Autodesk Fusion 360 part; units mm, degrees
(part 5 of 5)
  spline S157 degree 5 poles (17.2538, -21.1174) (17.2562, -21.1195) (17.2652, -21.1272) (17.281, -21.1406) (17.3036, -21.1597) (17.333, -21.1842) (17.3671, -21.2121) (17.4015, -21.2398) (17.4361, -21.2672) (17.4709, -21.2944) (17.506, -21.3214) (17.5413, -21.3481) (17.5769, -21.3747) (17.6126, -21.401) (17.6486, -21.4271) (17.6847, -21.4531) (17.7211, -21.4788) (17.7577, -21.5044) (17.7944, -21.5297) (17.8313, -21.5549) (17.8685, -21.5799) (17.9058, -21.6047) (17.9432, -21.6293) (17.9809, -21.6538) (18.0187, -21.6781) (18.0567, -21.7022) (18.0948, -21.7261) (18.1331, -21.7499) (18.1716, -21.7735) (18.2102, -21.7969) (18.249, -21.8202) (18.288, -21.8433) (18.3271, -21.8662) (18.3663, -21.889) (18.4057, -21.9116) (18.4452, -21.9341) (18.4849, -21.9564) (18.5247, -21.9785) (18.5646, -22.0005) (18.6047, -22.0224) (18.645, -22.0441) (18.6853, -22.0656) (18.7258, -22.087) (18.7664, -22.1083) (18.8072, -22.1294) (18.8481, -22.1503) (18.8891, -22.1711) (18.9302, -22.1918) (18.9715, -22.2123) (19.0129, -22.2326) (19.0544, -22.2529) (19.096, -22.2729) (19.1378, -22.2929) (19.1797, -22.3127) (19.2217, -22.3323) (19.2638, -22.3518) (19.306, -22.3712) (19.3483, -22.3904) (19.3908, -22.4095) (19.4334, -22.4284) (19.476, -22.4473) (19.5188, -22.4659) (19.5531, -22.4808) (19.5789, -22.4918) (19.5961, -22.4992) (19.6048, -22.5028) knots 0.13777296 0.13777296 0.13777296 0.13777296 0.13777296 0.13777296 0.14285714 0.15714286 0.17142857 0.18571429 0.2 0.21428571 0.22857143 0.24285714 0.25714286 0.27142857 0.28571429 0.3 0.31428571 0.32857143 0.34285714 0.35714286 0.37142857 0.38571429 0.4 0.41428571 0.42857143 0.44285714 0.45714286 0.47142857 0.48571429 0.5 0.51428571 0.52857143 0.54285714 0.55714286 0.57142857 0.58571429 0.6 0.61428571 0.62857143 0.64285714 0.65714286 0.67142857 0.68571429 0.7 0.71428571 0.72857143 0.74285714 0.75714286 0.77142857 0.78571429 0.8 0.81428571 0.82857143 0.84285714 0.85714286 0.87142857 0.88571429 0.9 0.91428571 0.92857143 0.94285714 0.95714286 0.97142857 0.98571429 1 1 1 1 1 1
  arc A79 (19.6048, -22.5028) -> (20.3303, -21.8495) centre (0, 0) ccw
  spline S158 degree 5 poles (20.3303, -21.8495) (20.3276, -21.8406) (20.3221, -21.8227) (20.3137, -21.7959) (20.3026, -21.7602) (20.2885, -21.7157) (20.2742, -21.6713) (20.2598, -21.627) (20.2453, -21.5828) (20.2306, -21.5387) (20.2158, -21.4946) (20.2008, -21.4507) (20.1856, -21.4069) (20.1703, -21.3632) (20.1548, -21.3196) (20.1392, -21.2761) (20.1235, -21.2327) (20.1075, -21.1894) (20.0915, -21.1462) (20.0752, -21.1031) (20.0588, -21.0602) (20.0423, -21.0173) (20.0255, -20.9746) (20.0087, -20.9319) (19.9916, -20.8894) (19.9744, -20.847) (19.957, -20.8048) (19.9395, -20.7626) (19.9218, -20.7206) (19.9039, -20.6787) (19.8859, -20.6369) (19.8677, -20.5952) (19.8493, -20.5537) (19.8307, -20.5123) (19.812, -20.471) (19.7931, -20.4299) (19.774, -20.3889) (19.7547, -20.348) (19.7353, -20.3073) (19.7157, -20.2667) (19.6958, -20.2263) (19.6758, -20.186) (19.6557, -20.1458) (19.6353, -20.1058) (19.6147, -20.066) (19.5939, -20.0263) (19.573, -19.9868) (19.5518, -19.9474) (19.5304, -19.9082) (19.5088, -19.8692) (19.487, -19.8303) (19.465, -19.7917) (19.4428, -19.7532) (19.4203, -19.7148) (19.3976, -19.6767) (19.3747, -19.6388) (19.3516, -19.6011) (19.3281, -19.5636) (19.3045, -19.5263) (19.2805, -19.4893) (19.2563, -19.4524) (19.235, -19.4206) (19.2185, -19.3961) (19.2068, -19.379) (19.2, -19.3692) (19.1982, -19.3667) knots -1 -1 -1 -1 -1 -1 -0.98571429 -0.97142857 -0.95714286 -0.94285714 -0.92857143 -0.91428571 -0.9 -0.88571429 -0.87142857 -0.85714286 -0.84285714 -0.82857143 -0.81428571 -0.8 -0.78571429 -0.77142857 -0.75714286 -0.74285714 -0.72857143 -0.71428571 -0.7 -0.68571429 -0.67142857 -0.65714286 -0.64285714 -0.62857143 -0.61428571 -0.6 -0.58571429 -0.57142857 -0.55714286 -0.54285714 -0.52857143 -0.51428571 -0.5 -0.48571429 -0.47142857 -0.45714286 -0.44285714 -0.42857143 -0.41428571 -0.4 -0.38571429 -0.37142857 -0.35714286 -0.34285714 -0.32857143 -0.31428571 -0.3 -0.28571429 -0.27142857 -0.25714286 -0.24285714 -0.22857143 -0.21428571 -0.2 -0.18571429 -0.17142857 -0.15714286 -0.14285714 -0.13777296 -0.13777296 -0.13777296 -0.13777296 -0.13777296 -0.13777296
  spline S159 degree 3 poles (19.221, -19.112) (19.2026, -19.1305) (19.188, -19.1523) (19.1681, -19.2004) (19.1629, -19.2262) (19.1627, -19.2726) (19.1657, -19.2928) (19.1778, -19.3316) (19.1867, -19.3499) (19.1982, -19.3667) knots 0 0 0 0 0.007813 0.007813 0.015626 0.015626 0.021719 0.021719 0.027811 0.027811 0.027811 0.027811
  arc A80 (19.221, -19.112) -> (19.7711, -18.5423) centre (0, 0) ccw
  spline S160 degree 3 poles (20.0249, -18.5107) (20.0029, -18.4966) (19.9785, -18.487) (19.9272, -18.4777) (19.9009, -18.478) (19.8556, -18.4877) (19.8365, -18.4949) (19.8011, -18.5148) (19.785, -18.5275) (19.7711, -18.5423) knots 0 0 0 0 0.007813 0.007813 0.015626 0.015626 0.021719 0.021719 0.027811 0.027811 0.027811 0.027811
  spline S161 degree 5 poles (20.0249, -18.5107) (20.0275, -18.5123) (20.0375, -18.5188) (20.055, -18.5299) (20.08, -18.5456) (20.1126, -18.5657) (20.1503, -18.5886) (20.1881, -18.6113) (20.2262, -18.6336) (20.2645, -18.6557) (20.303, -18.6775) (20.3417, -18.6991) (20.3806, -18.7204) (20.4197, -18.7415) (20.4589, -18.7624) (20.4983, -18.7831) (20.5379, -18.8035) (20.5777, -18.8237) (20.6176, -18.8437) (20.6577, -18.8635) (20.6979, -18.8831) (20.7383, -18.9025) (20.7788, -18.9216) (20.8195, -18.9406) (20.8603, -18.9594) (20.9013, -18.978) (20.9424, -18.9963) (20.9837, -19.0146) (21.0251, -19.0326) (21.0666, -19.0504) (21.1082, -19.068) (21.15, -19.0855) (21.1919, -19.1028) (21.2339, -19.1199) (21.2761, -19.1368) (21.3183, -19.1535) (21.3607, -19.1701) (21.4032, -19.1865) (21.4458, -19.2027) (21.4886, -19.2188) (21.5314, -19.2347) (21.5744, -19.2504) (21.6175, -19.2659) (21.6607, -19.2813) (21.704, -19.2965) (21.7474, -19.3116) (21.7909, -19.3265) (21.8345, -19.3412) (21.8782, -19.3558) (21.922, -19.3702) (21.966, -19.3844) (22.01, -19.3985) (22.0541, -19.4125) (22.0983, -19.4262) (22.1426, -19.4398) (22.1871, -19.4533) (22.2316, -19.4666) (22.2762, -19.4797) (22.3209, -19.4927) (22.3657, -19.5056) (22.4105, -19.5183) (22.4555, -19.5308) (22.4916, -19.5407) (22.5186, -19.5481) (22.5367, -19.5529) (22.5458, -19.5554) knots 0.13777296 0.13777296 0.13777296 0.13777296 0.13777296 0.13777296 0.14285714 0.15714286 0.17142857 0.18571429 0.2 0.21428571 0.22857143 0.24285714 0.25714286 0.27142857 0.28571429 0.3 0.31428571 0.32857143 0.34285714 0.35714286 0.37142857 0.38571429 0.4 0.41428571 0.42857143 0.44285714 0.45714286 0.47142857 0.48571429 0.5 0.51428571 0.52857143 0.54285714 0.55714286 0.57142857 0.58571429 0.6 0.61428571 0.62857143 0.64285714 0.65714286 0.67142857 0.68571429 0.7 0.71428571 0.72857143 0.74285714 0.75714286 0.77142857 0.78571429 0.8 0.81428571 0.82857143 0.84285714 0.85714286 0.87142857 0.88571429 0.9 0.91428571 0.92857143 0.94285714 0.95714286 0.97142857 0.98571429 1 1 1 1 1 1
  arc A81 (22.5458, -19.5554) -> (23.1733, -18.8075) centre (0, 0) ccw
  spline S162 degree 5 poles (23.1733, -18.8075) (23.1694, -18.799) (23.1614, -18.7821) (23.1495, -18.7567) (23.1334, -18.7229) (23.1133, -18.6808) (23.093, -18.6388) (23.0726, -18.5969) (23.052, -18.5551) (23.0313, -18.5135) (23.0105, -18.472) (22.9895, -18.4306) (22.9684, -18.3893) (22.9472, -18.3481) (22.9258, -18.3071) (22.9043, -18.2662) (22.8826, -18.2254) (22.8608, -18.1847) (22.8389, -18.1442) (22.8168, -18.1038) (22.7946, -18.0636) (22.7722, -18.0234) (22.7497, -17.9834) (22.7271, -17.9436) (22.7043, -17.9039) (22.6814, -17.8643) (22.6583, -17.8248) (22.635, -17.7855) (22.6117, -17.7464) (22.5881, -17.7073) (22.5644, -17.6685) (22.5406, -17.6298) (22.5166, -17.5912) (22.4925, -17.5528) (22.4682, -17.5145) (22.4438, -17.4764) (22.4191, -17.4385) (22.3944, -17.4007) (22.3695, -17.363) (22.3444, -17.3256) (22.3191, -17.2883) (22.2937, -17.2512) (22.2681, -17.2142) (22.2424, -17.1774) (22.2165, -17.1409) (22.1904, -17.1044) (22.1641, -17.0682) (22.1376, -17.0322) (22.111, -16.9964) (22.0842, -16.9607) (22.0572, -16.9253) (22.03, -16.89) (22.0027, -16.855) (21.9751, -16.8202) (21.9473, -16.7856) (21.9194, -16.7512) (21.8912, -16.7171) (21.8628, -16.6832) (21.8341, -16.6496) (21.8053, -16.6163) (21.7762, -16.5832) (21.7507, -16.5546) (21.7309, -16.5327) (21.7169, -16.5174) (21.7088, -16.5086) (21.7067, -16.5063) knots -1 -1 -1 -1 -1 -1 -0.98571429 -0.97142857 -0.95714286 -0.94285714 -0.92857143 -0.91428571 -0.9 -0.88571429 -0.87142857 -0.85714286 -0.84285714 -0.82857143 -0.81428571 -0.8 -0.78571429 -0.77142857 -0.75714286 -0.74285714 -0.72857143 -0.71428571 -0.7 -0.68571429 -0.67142857 -0.65714286 -0.64285714 -0.62857143 -0.61428571 -0.6 -0.58571429 -0.57142857 -0.55714286 -0.54285714 -0.52857143 -0.51428571 -0.5 -0.48571429 -0.47142857 -0.45714286 -0.44285714 -0.42857143 -0.41428571 -0.4 -0.38571429 -0.37142857 -0.35714286 -0.34285714 -0.32857143 -0.31428571 -0.3 -0.28571429 -0.27142857 -0.25714286 -0.24285714 -0.22857143 -0.21428571 -0.2 -0.18571429 -0.17142857 -0.15714286 -0.14285714 -0.13777296 -0.13777296 -0.13777296 -0.13777296 -0.13777296 -0.13777296
  spline S163 degree 3 poles (21.6938, -16.2509) (21.6782, -16.2718) (21.6668, -16.2955) (21.6537, -16.3459) (21.6522, -16.3721) (21.6585, -16.4181) (21.6643, -16.4377) (21.6816, -16.4744) (21.693, -16.4914) (21.7067, -16.5063) knots 0 0 0 0 0.007813 0.007813 0.015626 0.015626 0.021719 0.021719 0.027811 0.027811 0.027811 0.027811
  arc A82 (21.6938, -16.2509) -> (22.1593, -15.6102) centre (0, 0) ccw
  spline S164 degree 3 poles (22.4062, -15.5436) (22.3825, -15.5327) (22.3569, -15.5266) (22.3049, -15.5245) (22.2789, -15.5285) (22.2353, -15.5444) (22.2174, -15.5542) (22.1852, -15.5789) (22.171, -15.5936) (22.1593, -15.6102) knots 0 0 0 0 0.007813 0.007813 0.015626 0.015626 0.021719 0.021719 0.027811 0.027811 0.027811 0.027811
  spline S165 degree 5 poles (22.4062, -15.5436) (22.409, -15.5449) (22.4198, -15.5498) (22.4387, -15.5584) (22.4656, -15.5705) (22.5007, -15.5859) (22.5412, -15.6033) (22.5818, -15.6205) (22.6227, -15.6373) (22.6637, -15.6539) (22.7048, -15.6701) (22.7461, -15.6861) (22.7876, -15.7018) (22.8293, -15.7173) (22.871, -15.7325) (22.9129, -15.7475) (22.955, -15.7622) (22.9972, -15.7767) (23.0395, -15.7909) (23.0819, -15.8049) (23.1245, -15.8187) (23.1672, -15.8323) (23.21, -15.8456) (23.2529, -15.8588) (23.296, -15.8717) (23.3391, -15.8844) (23.3824, -15.8969) (23.4258, -15.9091) (23.4693, -15.9212) (23.5128, -15.9331) (23.5565, -15.9448) (23.6003, -15.9562) (23.6442, -15.9675) (23.6882, -15.9786) (23.7323, -15.9895) (23.7765, -16.0002) (23.8208, -16.0107) (23.8652, -16.021) (23.9096, -16.0312) (23.9542, -16.0411) (23.9989, -16.0509) (24.0436, -16.0605) (24.0884, -16.0699) (24.1333, -16.0791) (24.1783, -16.0881) (24.2234, -16.097) (24.2685, -16.1057) (24.3138, -16.1142) (24.3591, -16.1226) (24.4045, -16.1307) (24.45, -16.1387) (24.4955, -16.1465) (24.5412, -16.1542) (24.5869, -16.1617) (24.6327, -16.169) (24.6785, -16.1761) (24.7244, -16.1831) (24.7704, -16.1899) (24.8165, -16.1966) (24.8627, -16.2031) (24.9089, -16.2094) (24.9551, -16.2155) (24.9922, -16.2203) (25.0201, -16.2238) (25.0386, -16.2262) (25.0479, -16.2273) knots 0.13777296 0.13777296 0.13777296 0.13777296 0.13777296 0.13777296 0.14285714 0.15714286 0.17142857 0.18571429 0.2 0.21428571 0.22857143 0.24285714 0.25714286 0.27142857 0.28571429 0.3 0.31428571 0.32857143 0.34285714 0.35714286 0.37142857 0.38571429 0.4 0.41428571 0.42857143 0.44285714 0.45714286 0.47142857 0.48571429 0.5 0.51428571 0.52857143 0.54285714 0.55714286 0.57142857 0.58571429 0.6 0.61428571 0.62857143 0.64285714 0.65714286 0.67142857 0.68571429 0.7 0.71428571 0.72857143 0.74285714 0.75714286 0.77142857 0.78571429 0.8 0.81428571 0.82857143 0.84285714 0.85714286 0.87142857 0.88571429 0.9 0.91428571 0.92857143 0.94285714 0.95714286 0.97142857 0.98571429 1 1 1 1 1 1
  arc A83 (25.0479, -16.2273) -> (25.5653, -15.3993) centre (0, 0) ccw
  spline S166 degree 5 poles (25.5653, -15.3993) (25.5602, -15.3915) (25.55, -15.3758) (25.5346, -15.3523) (25.514, -15.3211) (25.4882, -15.2822) (25.4623, -15.2435) (25.4362, -15.2048) (25.4101, -15.1663) (25.3838, -15.128) (25.3574, -15.0898) (25.3308, -15.0517) (25.3042, -15.0137) (25.2774, -14.9759) (25.2506, -14.9383) (25.2236, -14.9008) (25.1964, -14.8634) (25.1692, -14.8262) (25.1418, -14.7891) (25.1143, -14.7522) (25.0867, -14.7154) (25.059, -14.6787) (25.0312, -14.6423) (25.0032, -14.6059) (24.9751, -14.5698) (24.9469, -14.5338) (24.9185, -14.4979) (24.89, -14.4622) (24.8614, -14.4267) (24.8327, -14.3914) (24.8038, -14.3562) (24.7748, -14.3211) (24.7457, -14.2863) (24.7165, -14.2516) (24.6871, -14.2171) (24.6576, -14.1828) (24.6279, -14.1486) (24.5981, -14.1146) (24.5682, -14.0808) (24.5382, -14.0472) (24.508, -14.0138) (24.4776, -13.9806) (24.4472, -13.9476) (24.4165, -13.9147) (24.3858, -13.8821) (24.3549, -13.8497) (24.3238, -13.8175) (24.2926, -13.7855) (24.2613, -13.7537) (24.2298, -13.7221) (24.1981, -13.6908) (24.1663, -13.6597) (24.1343, -13.6288) (24.1021, -13.5982) (24.0698, -13.5678) (24.0374, -13.5376) (24.0047, -13.5077) (23.9719, -13.4782) (23.9388, -13.4489) (23.9056, -13.4198) (23.8722, -13.3911) (23.8429, -13.3663) (23.8203, -13.3474) (23.8043, -13.3342) (23.7951, -13.3267) (23.7927, -13.3247) knots -1 -1 -1 -1 -1 -1 -0.98571429 -0.97142857 -0.95714286 -0.94285714 -0.92857143 -0.91428571 -0.9 -0.88571429 -0.87142857 -0.85714286 -0.84285714 -0.82857143 -0.81428571 -0.8 -0.78571429 -0.77142857 -0.75714286 -0.74285714 -0.72857143 -0.71428571 -0.7 -0.68571429 -0.67142857 -0.65714286 -0.64285714 -0.62857143 -0.61428571 -0.6 -0.58571429 -0.57142857 -0.55714286 -0.54285714 -0.52857143 -0.51428571 -0.5 -0.48571429 -0.47142857 -0.45714286 -0.44285714 -0.42857143 -0.41428571 -0.4 -0.38571429 -0.37142857 -0.35714286 -0.34285714 -0.32857143 -0.31428571 -0.3 -0.28571429 -0.27142857 -0.25714286 -0.24285714 -0.22857143 -0.21428571 -0.2 -0.18571429 -0.17142857 -0.15714286 -0.14285714 -0.13777296 -0.13777296 -0.13777296 -0.13777296 -0.13777296 -0.13777296
  spline S167 degree 3 poles (23.7444, -13.0736) (23.7318, -13.0964) (23.7238, -13.1215) (23.7179, -13.1732) (23.72, -13.1994) (23.7326, -13.244) (23.7411, -13.2626) (23.7634, -13.2966) (23.777, -13.3118) (23.7927, -13.3247) knots 0 0 0 0 0.007813 0.007813 0.015626 0.015626 0.021719 0.021719 0.027811 0.027811 0.027811 0.027811
  arc A84 (23.7444, -13.0736) -> (24.1162, -12.3743) centre (0, 0) ccw
  spline S168 degree 3 poles (24.3514, -12.274) (24.3264, -12.2665) (24.3002, -12.264) (24.2484, -12.2692) (24.2232, -12.2768) (24.1823, -12.2986) (24.1659, -12.3108) (24.1374, -12.3397) (24.1255, -12.3562) (24.1162, -12.3743) knots 0 0 0 0 0.007813 0.007813 0.015626 0.015626 0.021719 0.021719 0.027811 0.027811 0.027811 0.027811
  spline S169 degree 5 poles (24.3514, -12.274) (24.3544, -12.2749) (24.3658, -12.2783) (24.3856, -12.2841) (24.414, -12.2923) (24.4509, -12.3027) (24.4934, -12.3144) (24.536, -12.3257) (24.5788, -12.3367) (24.6217, -12.3474) (24.6647, -12.3577) (24.7079, -12.3678) (24.7511, -12.3776) (24.7945, -12.3871) (24.838, -12.3963) (24.8816, -12.4053) (24.9253, -12.4141) (24.9691, -12.4225) (25.0129, -12.4308) (25.0569, -12.4387) (25.101, -12.4465) (25.1452, -12.454) (25.1894, -12.4612) (25.2337, -12.4682) (25.2782, -12.475) (25.3227, -12.4816) (25.3673, -12.4879) (25.4119, -12.4941) (25.4567, -12.5) (25.5015, -12.5057) (25.5464, -12.5112) (25.5913, -12.5164) (25.6364, -12.5215) (25.6815, -12.5263) (25.7267, -12.531) (25.7719, -12.5354) (25.8172, -12.5397) (25.8626, -12.5437) (25.9081, -12.5476) (25.9536, -12.5512) (25.9991, -12.5547) (26.0448, -12.558) (26.0905, -12.561) (26.1362, -12.5639) (26.182, -12.5666) (26.2279, -12.5691) (26.2738, -12.5714) (26.3198, -12.5736) (26.3659, -12.5755) (26.412, -12.5773) (26.4581, -12.5789) (26.5043, -12.5803) (26.5506, -12.5815) (26.5969, -12.5826) (26.6432, -12.5834) (26.6896, -12.5841) (26.7361, -12.5846) (26.7826, -12.585) (26.8291, -12.5852) (26.8757, -12.5852) (26.9224, -12.585) (26.969, -12.5846) (27.0064, -12.5842) (27.0345, -12.5838) (27.0532, -12.5835) (27.0626, -12.5834) knots 0.13777296 0.13777296 0.13777296 0.13777296 0.13777296 0.13777296 0.14285714 0.15714286 0.17142857 0.18571429 0.2 0.21428571 0.22857143 0.24285714 0.25714286 0.27142857 0.28571429 0.3 0.31428571 0.32857143 0.34285714 0.35714286 0.37142857 0.38571429 0.4 0.41428571 0.42857143 0.44285714 0.45714286 0.47142857 0.48571429 0.5 0.51428571 0.52857143 0.54285714 0.55714286 0.57142857 0.58571429 0.6 0.61428571 0.62857143 0.64285714 0.65714286 0.67142857 0.68571429 0.7 0.71428571 0.72857143 0.74285714 0.75714286 0.77142857 0.78571429 0.8 0.81428571 0.82857143 0.84285714 0.85714286 0.87142857 0.88571429 0.9 0.91428571 0.92857143 0.94285714 0.95714286 0.97142857 0.98571429 1 1 1 1 1 1
  arc A85 (27.0626, -12.5834) -> (27.4597, -11.6915) centre (0, 0) ccw
  spline S170 degree 5 poles (27.4597, -11.6915) (27.4535, -11.6844) (27.4412, -11.6703) (27.4227, -11.6492) (27.398, -11.6211) (27.367, -11.5862) (27.336, -11.5514) (27.3048, -11.5168) (27.2735, -11.4823) (27.2421, -11.448) (27.2107, -11.4138) (27.1791, -11.3798) (27.1474, -11.346) (27.1157, -11.3122) (27.0838, -11.2787) (27.0519, -11.2453) (27.0198, -11.2121) (26.9876, -11.179) (26.9554, -11.1461) (26.923, -11.1133) (26.8906, -11.0808) (26.858, -11.0484) (26.8254, -11.0161) (26.7926, -10.984) (26.7597, -10.9521) (26.7268, -10.9204) (26.6937, -10.8889) (26.6606, -10.8575) (26.6273, -10.8263) (26.5939, -10.7953) (26.5604, -10.7644) (26.5268, -10.7338) (26.4932, -10.7033) (26.4594, -10.673) (26.4255, -10.6429) (26.3915, -10.6131) (26.3574, -10.5834) (26.3231, -10.5539) (26.2888, -10.5246) (26.2544, -10.4955) (26.2198, -10.4666) (26.1851, -10.4379) (26.1504, -10.4094) (26.1155, -10.3812) (26.0805, -10.3532) (26.0454, -10.3254) (26.0101, -10.2978) (25.9748, -10.2704) (25.9393, -10.2433) (25.9037, -10.2165) (25.868, -10.1898) (25.8321, -10.1634) (25.7962, -10.1373) (25.7601, -10.1114) (25.7239, -10.0858) (25.6875, -10.0605) (25.651, -10.0355) (25.6144, -10.0108) (25.5776, -9.9863) (25.5406, -9.9622) (25.5036, -9.9384) (25.4711, -9.918) (25.4461, -9.9024) (25.4284, -9.8915) (25.4183, -9.8853) (25.4156, -9.8837) knots -1 -1 -1 -1 -1 -1 -0.98571429 -0.97142857 -0.95714286 -0.94285714 -0.92857143 -0.91428571 -0.9 -0.88571429 -0.87142857 -0.85714286 -0.84285714 -0.82857143 -0.81428571 -0.8 -0.78571429 -0.77142857 -0.75714286 -0.74285714 -0.72857143 -0.71428571 -0.7 -0.68571429 -0.67142857 -0.65714286 -0.64285714 -0.62857143 -0.61428571 -0.6 -0.58571429 -0.57142857 -0.55714286 -0.54285714 -0.52857143 -0.51428571 -0.5 -0.48571429 -0.47142857 -0.45714286 -0.44285714 -0.42857143 -0.41428571 -0.4 -0.38571429 -0.37142857 -0.35714286 -0.34285714 -0.32857143 -0.31428571 -0.3 -0.28571429 -0.27142857 -0.25714286 -0.24285714 -0.22857143 -0.21428571 -0.2 -0.18571429 -0.17142857 -0.15714286 -0.14285714 -0.13777296 -0.13777296 -0.13777296 -0.13777296 -0.13777296 -0.13777296
  spline S171 degree 3 poles (25.3328, -9.6418) (25.3235, -9.6661) (25.3191, -9.692) (25.3204, -9.7441) (25.3262, -9.7698) (25.3449, -9.8122) (25.3559, -9.8294) (25.3826, -9.86) (25.3982, -9.8731) (25.4156, -9.8837) knots 0 0 0 0 0.007813 0.007813 0.015626 0.015626 0.021719 0.021719 0.027811 0.027811 0.027811 0.027811
  arc A86 (25.3328, -9.6418) -> (25.6037, -8.8976) centre (0, 0) ccw
  spline S172 degree 3 poles (25.8226, -8.7655) (25.7968, -8.7616) (25.7706, -8.7627) (25.72, -8.775) (25.6961, -8.7861) (25.6586, -8.8133) (25.6441, -8.8277) (25.6199, -8.8603) (25.6103, -8.8784) (25.6037, -8.8976) knots 0 0 0 0 0.007813 0.007813 0.015626 0.015626 0.021719 0.021719 0.027811 0.027811 0.027811 0.027811
  spline S173 degree 5 poles (25.8226, -8.7655) (25.8257, -8.7659) (25.8375, -8.7677) (25.8579, -8.7708) (25.8872, -8.7749) (25.9252, -8.7801) (25.9689, -8.7857) (26.0127, -8.791) (26.0565, -8.7959) (26.1005, -8.8005) (26.1445, -8.8048) (26.1887, -8.8088) (26.2329, -8.8124) (26.2772, -8.8158) (26.3215, -8.8189) (26.3659, -8.8218) (26.4104, -8.8243) (26.4549, -8.8266) (26.4995, -8.8287) (26.5442, -8.8304) (26.5889, -8.832) (26.6337, -8.8332) (26.6785, -8.8343) (26.7234, -8.835) (26.7683, -8.8356) (26.8133, -8.8359) (26.8584, -8.836) (26.9035, -8.8358) (26.9486, -8.8355) (26.9938, -8.8349) (27.039, -8.834) (27.0842, -8.833) (27.1295, -8.8317) (27.1749, -8.8303) (27.2203, -8.8286) (27.2657, -8.8267) (27.3112, -8.8246) (27.3567, -8.8223) (27.4022, -8.8198) (27.4478, -8.817) (27.4934, -8.8141) (27.539, -8.811) (27.5847, -8.8077) (27.6304, -8.8042) (27.6762, -8.8005) (27.722, -8.7966) (27.7678, -8.7925) (27.8136, -8.7882) (27.8595, -8.7837) (27.9053, -8.7791) (27.9513, -8.7742) (27.9972, -8.7692) (28.0432, -8.7639) (28.0892, -8.7585) (28.1352, -8.7529) (28.1813, -8.7472) (28.2273, -8.7412) (28.2734, -8.7351) (28.3195, -8.7288) (28.3657, -8.7223) (28.4118, -8.7156) (28.458, -8.7088) (28.495, -8.7032) (28.5227, -8.6989) (28.5412, -8.696) (28.5505, -8.6945) knots 0.13777296 0.13777296 0.13777296 0.13777296 0.13777296 0.13777296 0.14285714 0.15714286 0.17142857 0.18571429 0.2 0.21428571 0.22857143 0.24285714 0.25714286 0.27142857 0.28571429 0.3 0.31428571 0.32857143 0.34285714 0.35714286 0.37142857 0.38571429 0.4 0.41428571 0.42857143 0.44285714 0.45714286 0.47142857 0.48571429 0.5 0.51428571 0.52857143 0.54285714 0.55714286 0.57142857 0.58571429 0.6 0.61428571 0.62857143 0.64285714 0.65714286 0.67142857 0.68571429 0.7 0.71428571 0.72857143 0.74285714 0.75714286 0.77142857 0.78571429 0.8 0.81428571 0.82857143 0.84285714 0.85714286 0.87142857 0.88571429 0.9 0.91428571 0.92857143 0.94285714 0.95714286 0.97142857 0.98571429 1 1 1 1 1 1
  arc A87 (28.5505, -8.6945) -> (28.8196, -7.756) centre (0, 0) ccw
  spline S174 degree 5 poles (28.8196, -7.756) (28.8125, -7.7499) (28.7984, -7.7377) (28.7771, -7.7193) (28.7487, -7.695) (28.7132, -7.6647) (28.6776, -7.6346) (28.6419, -7.6046) (28.6061, -7.5749) (28.5703, -7.5452) (28.5344, -7.5158) (28.4984, -7.4865) (28.4623, -7.4573) (28.4262, -7.4284) (28.3899, -7.3996) (28.3536, -7.371) (28.3173, -7.3425) (28.2808, -7.3142) (28.2443, -7.2861) (28.2077, -7.2582) (28.171, -7.2305) (28.1343, -7.2029) (28.0974, -7.1755) (28.0605, -7.1483) (28.0236, -7.1213) (27.9865, -7.0945) (27.9494, -7.0678) (27.9122, -7.0414) (27.8749, -7.0151) (27.8375, -6.989) (27.8001, -6.9632) (27.7625, -6.9375) (27.7249, -6.912) (27.6873, -6.8867) (27.6495, -6.8617) (27.6117, -6.8368) (27.5738, -6.8121) (27.5358, -6.7877) (27.4977, -6.7634) (27.4595, -6.7394) (27.4213, -6.7156) (27.383, -6.6921) (27.3446, -6.6687) (27.3061, -6.6456) (27.2676, -6.6227) (27.2289, -6.6001) (27.1902, -6.5777) (27.1514, -6.5555) (27.1125, -6.5336) (27.0735, -6.5119) (27.0344, -6.4905) (26.9952, -6.4694) (26.956, -6.4485) (26.9166, -6.4279) (26.8772, -6.4076) (26.8377, -6.3876) (26.798, -6.3679) (26.7583, -6.3485) (26.7185, -6.3294) (26.6786, -6.3107) (26.6385, -6.2923) (26.6036, -6.2765) (26.5766, -6.2646) (26.5576, -6.2563) (26.5467, -6.2516) (26.5438, -6.2503) knots -1 -1 -1 -1 -1 -1 -0.98571429 -0.97142857 -0.95714286 -0.94285714 -0.92857143 -0.91428571 -0.9 -0.88571429 -0.87142857 -0.85714286 -0.84285714 -0.82857143 -0.81428571 -0.8 -0.78571429 -0.77142857 -0.75714286 -0.74285714 -0.72857143 -0.71428571 -0.7 -0.68571429 -0.67142857 -0.65714286 -0.64285714 -0.62857143 -0.61428571 -0.6 -0.58571429 -0.57142857 -0.55714286 -0.54285714 -0.52857143 -0.51428571 -0.5 -0.48571429 -0.47142857 -0.45714286 -0.44285714 -0.42857143 -0.41428571 -0.4 -0.38571429 -0.37142857 -0.35714286 -0.34285714 -0.32857143 -0.31428571 -0.3 -0.28571429 -0.27142857 -0.25714286 -0.24285714 -0.22857143 -0.21428571 -0.2 -0.18571429 -0.17142857 -0.15714286 -0.14285714 -0.13777296 -0.13777296 -0.13777296 -0.13777296 -0.13777296 -0.13777296
  spline S175 degree 3 poles (26.4281, -6.0223) (26.4223, -6.0477) (26.4216, -6.074) (26.4301, -6.1254) (26.4394, -6.15) (26.4638, -6.1894) (26.4771, -6.2049) (26.5078, -6.2314) (26.5251, -6.2423) (26.5438, -6.2503) knots 0 0 0 0 0.007813 0.007813 0.015626 0.015626 0.021719 0.021719 0.027811 0.027811 0.027811 0.027811
  arc A88 (26.4281, -6.0223) -> (26.5928, -5.2476) centre (0, 0) ccw
  spline S176 degree 3 poles (26.7912, -5.0864) (26.7652, -5.0861) (26.7393, -5.0909) (26.6909, -5.1101) (26.6688, -5.1244) (26.6355, -5.1566) (26.6231, -5.1728) (26.6037, -5.2085) (26.5967, -5.2277) (26.5928, -5.2476) knots 0 0 0 0 0.007813 0.007813 0.015626 0.015626 0.021719 0.021719 0.027811 0.027811 0.027811 0.027811
  spline S177 degree 5 poles (26.7912, -5.0864) (26.7943, -5.0864) (26.8062, -5.0865) (26.827, -5.0867) (26.8565, -5.0867) (26.8948, -5.0866) (26.9389, -5.086) (26.983, -5.0852) (27.0271, -5.0839) (27.0713, -5.0824) (27.1155, -5.0805) (27.1598, -5.0783) (27.204, -5.0758) (27.2484, -5.073) (27.2927, -5.0699) (27.3371, -5.0665) (27.3815, -5.0628) (27.4259, -5.0589) (27.4704, -5.0547) (27.5148, -5.0503) (27.5593, -5.0455) (27.6038, -5.0406) (27.6484, -5.0353) (27.6929, -5.0299) (27.7375, -5.0242) (27.7821, -5.0182) (27.8267, -5.012) (27.8713, -5.0056) (27.916, -4.999) (27.9606, -4.9921) (28.0053, -4.985) (28.05, -4.9776) (28.0947, -4.9701) (28.1394, -4.9623) (28.1841, -4.9543) (28.2288, -4.9461) (28.2735, -4.9377) (28.3183, -4.9291) (28.363, -4.9203) (28.4078, -4.9112) (28.4525, -4.902) (28.4973, -4.8926) (28.5421, -4.8829) (28.5868, -4.8731) (28.6316, -4.863) (28.6764, -4.8528) (28.7212, -4.8424) (28.766, -4.8318) (28.8108, -4.8209) (28.8556, -4.8099) (28.9004, -4.7987) (28.9452, -4.7874) (28.99, -4.7758) (29.0348, -4.764) (29.0796, -4.7521) (29.1244, -4.74) (29.1692, -4.7277) (29.214, -4.7152) (29.2588, -4.7025) (29.3035, -4.6897) (29.3483, -4.6766) (29.3931, -4.6634) (29.4289, -4.6527) (29.4558, -4.6446) (29.4737, -4.6392) (29.4827, -4.6365) knots 0.13777296 0.13777296 0.13777296 0.13777296 0.13777296 0.13777296 0.14285714 0.15714286 0.17142857 0.18571429 0.2 0.21428571 0.22857143 0.24285714 0.25714286 0.27142857 0.28571429 0.3 0.31428571 0.32857143 0.34285714 0.35714286 0.37142857 0.38571429 0.4 0.41428571 0.42857143 0.44285714 0.45714286 0.47142857 0.48571429 0.5 0.51428571 0.52857143 0.54285714 0.55714286 0.57142857 0.58571429 0.6 0.61428571 0.62857143 0.64285714 0.65714286 0.67142857 0.68571429 0.7 0.71428571 0.72857143 0.74285714 0.75714286 0.77142857 0.78571429 0.8 0.81428571 0.82857143 0.84285714 0.85714286 0.87142857 0.88571429 0.9 0.91428571 0.92857143 0.94285714 0.95714286 0.97142857 0.98571429 1 1 1 1 1 1
  arc A89 (29.4827, -4.6365) -> (29.6185, -3.6697) centre (0, 0) ccw
  spline S178 degree 5 poles (29.6185, -3.6697) (29.6107, -3.6646) (29.595, -3.6544) (29.5714, -3.6392) (29.5399, -3.619) (29.5005, -3.594) (29.461, -3.5691) (29.4215, -3.5445) (29.3819, -3.5199) (29.3423, -3.4956) (29.3027, -3.4714) (29.2629, -3.4474) (29.2232, -3.4236) (29.1833, -3.3999) (29.1435, -3.3765) (29.1035, -3.3532) (29.0636, -3.3301) (29.0235, -3.3071) (28.9835, -3.2844) (28.9433, -3.2618) (28.9032, -3.2395) (28.8629, -3.2173) (28.8226, -3.1953) (28.7823, -3.1735) (28.7419, -3.1519) (28.7015, -3.1305) (28.661, -3.1092) (28.6205, -3.0882) (28.5799, -3.0674) (28.5393, -3.0468) (28.4986, -3.0264) (28.4579, -3.0062) (28.4171, -2.9862) (28.3763, -2.9664) (28.3354, -2.9468) (28.2945, -2.9275) (28.2535, -2.9083) (28.2125, -2.8894) (28.1714, -2.8707) (28.1303, -2.8522) (28.0891, -2.834) (28.0479, -2.816) (28.0066, -2.7982) (27.9653, -2.7806) (27.9239, -2.7633) (27.8825, -2.7463) (27.841, -2.7295) (27.7995, -2.713) (27.7579, -2.6967) (27.7163, -2.6807) (27.6746, -2.6649) (27.6329, -2.6494) (27.5911, -2.6342) (27.5493, -2.6193) (27.5074, -2.6047) (27.4655, -2.5904) (27.4235, -2.5764) (27.3814, -2.5627) (27.3393, -2.5493) (27.2972, -2.5364) (27.255, -2.5237) (27.2182, -2.513) (27.1898, -2.5049) (27.1698, -2.4993) (27.1584, -2.4962) (27.1553, -2.4953) knots -1 -1 -1 -1 -1 -1 -0.98571429 -0.97142857 -0.95714286 -0.94285714 -0.92857143 -0.91428571 -0.9 -0.88571429 -0.87142857 -0.85714286 -0.84285714 -0.82857143 -0.81428571 -0.8 -0.78571429 -0.77142857 -0.75714286 -0.74285714 -0.72857143 -0.71428571 -0.7 -0.68571429 -0.67142857 -0.65714286 -0.64285714 -0.62857143 -0.61428571 -0.6 -0.58571429 -0.57142857 -0.55714286 -0.54285714 -0.52857143 -0.51428571 -0.5 -0.48571429 -0.47142857 -0.45714286 -0.44285714 -0.42857143 -0.41428571 -0.4 -0.38571429 -0.37142857 -0.35714286 -0.34285714 -0.32857143 -0.31428571 -0.3 -0.28571429 -0.27142857 -0.25714286 -0.24285714 -0.22857143 -0.21428571 -0.2 -0.18571429 -0.17142857 -0.15714286 -0.14285714 -0.13777296 -0.13777296 -0.13777296 -0.13777296 -0.13777296 -0.13777296
  spline S179 degree 3 poles (27.0091, -2.2856) (27.0069, -2.3116) (27.0098, -2.3377) (27.0254, -2.3874) (27.038, -2.4105) (27.0677, -2.4461) (27.083, -2.4596) (27.1171, -2.4816) (27.1358, -2.4899) (27.1553, -2.4953) knots 0 0 0 0 0.007813 0.007813 0.015626 0.015626 0.021719 0.021719 0.027811 0.027811 0.027811 0.027811
  circle A90 centre (0, 0) radius 2.5
  circle A91 centre (0, 0) radius 33.0715
  dimension "d9" = 66.143
  constraint coincident A0.centre A1.centre
  measures "d9" diameter of A91
extrude "Extrude3" add sketch "Sketch4" along normal blind 3 separate body contours A91 makes body 2
hidden bodies 1
named bodies: "Spur Gear (45 teeth)"
